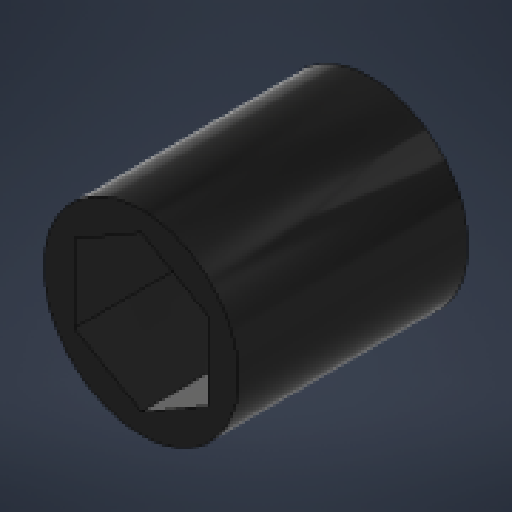
# Autodesk Inventor part: 3DPRINT,TURRET,HEX,SPACER
Saved by Autodesk Inventor 2026 (Build 300175000, 175)
## iProperties
Created: 2026-02-09
Part Number: 3DPRINT,TURRET,HEX,SPACER
Material: ABS Plastic
Document SubType Name: Modeling
Designer: littl
Density: 1.06 g/cm^3
Appearance: Smooth - Black
Author: littl
Autodesk Inventor part; units mm, degrees
ref_plane "YZ Plane" through (0, 0, 0) normal (1, 0, 0) x (0, 1, 0)
ref_plane "XZ Plane" through (0, 0, 0) normal (0, 1, 0) x (-1, 0, 0)
ref_plane "XY Plane" through (0, 0, 0) normal (0, 0, 1) x (1, 0, 0)
sketch "Sketch1" plane through (0, 0, 0) normal (0, 0, 1) x (1, 0, 0)
  line L0 (-6.985, -4.0328) -> (-6.985, 4.0328)
  line L1 (-6.985, 4.0328) -> (0, 8.0656)
  line L2 (0, 8.0656) -> (6.985, 4.0328)
  line L3 (6.985, 4.0328) -> (6.985, -4.0328)
  line L4 (6.985, -4.0328) -> (0, -8.0656)
  line L5 (0, -8.0656) -> (-6.985, -4.0328)
  circle A0 centre (0, 0) radius 10.16
  dimension "d0" = 13.97
  dimension "d1" = 20.32
  constraints: 12 end point, 2 coincident, 1 centre point, 1 vertical, 13 other
  measures "d0" distance between parallel lines of L3 L0
  measures "d1" diameter of A0
extrude "Extrusion1" add sketch "Sketch1" along normal blind 23.876
body "Solid1"
